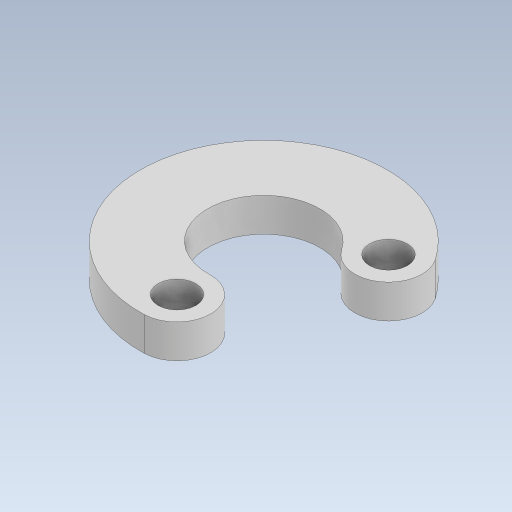
# Autodesk Inventor part: Tensioner2
Saved by Autodesk Inventor 2023 (Build 270158000, 158)
## iProperties
Created: 2022-09-14
Part Number: Tensioner2
Material: Generic
Document SubType Name: Modeling
Designer: Dave
Density: 1 g/cm^3
Appearance: Default
Author: Dave
Autodesk Inventor part; units mm, degrees
ref_plane "YZ Plane" through (0, 0, 0) normal (1, 0, 0) x (0, 1, 0)
ref_plane "XZ Plane" through (0, 0, 0) normal (0, 1, 0) x (-1, 0, 0)
ref_plane "XY Plane" through (0, 0, 0) normal (0, 0, 1) x (1, 0, 0)
sketch "Sketch1" plane through (0, 0, 0) normal (0, 1, 0) x (-1, 0, 0)
  arc A0 (6, 0) -> (-6, 0) centre (0, 0) ccw
  line L0 (6, 0) -> (6, -12.3)
  line L1 (4.2426, -16.5426) -> (-8.4574, -29.2426)
  line L2 (-16.9426, -20.7574) -> (-6, -9.8147)
  line L3 (-6, -9.8147) -> (-6, 0)
  arc A1 (-16.9426, -20.7574) -> (-8.4574, -29.2426) centre (-12.7, -25) ccw
  arc A2 (4.2426, -16.5426) -> (6, -12.3) centre (0, -12.3) ccw
  line L4 (0, 0) -> (-12.7, -25) construction
  circle A3 centre (0, 0) radius 6
  circle A4 centre (-12.7, -25) radius 6
  arc A5 (-7.7414, -21.6218) -> (0.1961, -5.9968) centre (0.5229, -15.9915) ccw
  arc A6 (-17.6586, -28.3782) -> (-0.1961, 5.9968) centre (0.5229, -15.9915) ccw
  point P0 (6, -14.7853)
  point P1 (-16.9426, -20.7574)
  point P2 (-17.6586, -28.3782)
  point P3 (-0.1961, 5.9968)
  point P4 (-6, 0)
  dimension "d0" = 12
  dimension "d1" = 12.7
  dimension "d2" = 25
  dimension "d3" = 135
  dimension "d6" = 6
  dimension "d14" = 10
  constraints: 14 point on circle, 10 end point, 10 tangent, 7 centre point, 4 coincident, 3 equal radius, 2 parallel, 2 point on line, 1 concentric, 1 vertical
  measures "d0" diameter of A0
  measures "d1" horizontal distance of point (0, 0) A1.centre
  measures "d2" vertical distance of A1.centre point (0, 0)
  measures "d3" angle of L3 L2
  measures "d6" radius of A2
  measures "d14" radius of A5
extrude "Extrusion1" add sketch "Sketch1" along normal blind 6 contours A3 A0 | A0 A6 A1 L1 A5 L0 | L0 A5 A3 | A1 A4 | L1 A4 A5
sketch "Sketch2" plane through (0, 6, 0) normal (0, 1, 0) x (1, 0, 0)
  arc A0 (7.7414, 21.6218) -> (17.6586, 28.3782) centre (12.7, 25) ccw projected
  point P0 (0, 0)
  point P1 (16.9426, 20.7574)
  point P2 (8.4574, 29.2426)
hole "Hole1" at (0, 6, 0) at (12.7, 6, -25) direction (0, -1, 0) diameter 6.7564 depth 12.7 tip angle 118 clearance for "Flat Head Machine Screw (82)" size "1/4" standard "Ansi Unified Screw Threads"
body "Solid1"
